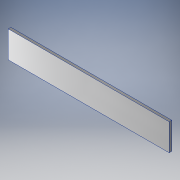
# Autodesk Inventor part: Frame Bottom Front
Saved by Autodesk Inventor 2019 (Build 230136000, 136)
## iProperties
Created: 2018-10-20
Part Number: Frame Bottom Front
Material: Aluminum 6061
Document SubType Name: Modeling
Designer: LillaHunden
Density: 2.7 g/cm^3
Appearance: Aluminum - Flat
Author: LillaHunden
Autodesk Inventor part; units mm, degrees
ref_plane "YZ Plane" through (0, 0, 0) normal (1, 0, 0) x (0, 1, 0)
ref_plane "XZ Plane" through (0, 0, 0) normal (0, 1, 0) x (-1, 0, 0)
ref_plane "XY Plane" through (0, 0, 0) normal (0, 0, 1) x (1, 0, 0)
sketch "Sketch1" plane through (0, 0, 0) normal (0, 0, 1) x (1, 0, 0)
  line L0 (288, 5.1258) -> (250.2, 5.1258) construction
  line L1 (0, 0) -> (300, 0) construction
  line L2 (300, 0) -> (300, 10) construction
  line L3 (-40, 10) -> (300, 10) construction
  line L4 (-40, 0) -> (-40, 10) construction
  line L5 (300, 0) -> (-40, 0)
  line L6 (-40, 0) -> (-40, 50)
  line L7 (-40, 50) -> (300, 50)
  line L8 (300, 50) -> (300, 0)
  line L9 (-40, 0) -> (-40, 10) projected
  dimension "d1" = 50
  constraints: 8 end point, 2 parallel, 1 horizontal, 1 perpendicular
  measures "d1" distance of L5.end L6.end
extrude "Extrusion1" add sketch "Sketch1" along normal blind 5
body "Solid1"
